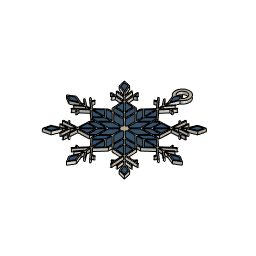
Snowflake 5 (Autodesk Fusion 360 design; units mm, degrees)
Autodesk Fusion 360 part; units mm, degrees
(part 1 of 2)
sketch "Sketch1" plane through (0, 0, 0) normal (0, 0, 1) x (1, 0, 0)
  line L0 (-4.9, 4.9) -> (4.9, 4.9)
  line L1 (4.9, 4.9) -> (4.9, -4.9)
  line L2 (4.9, -4.9) -> (-4.9, -4.9)
  line L3 (-4.9, -4.9) -> (-4.9, 4.9)
  line L4 (0, 4.9) -> (0, 0) construction
  line L5 (0, 0) -> (4.9, 0) construction
  dimension "d460" = 9.8
  constraint horizontal L0
  constraint vertical L1
  constraint vertical L3
  constraint horizontal L2
  constraint midpoint L0 L4.start
  constraint coincident L4.end L5.start
  constraint midpoint L1 L5.end
  constraint vertical L4
  constraint horizontal L5
  constraint equal L1 L2
  measures "d460" distance of L1.end L2.end
extrude "Extrude1" add sketch "Sketch1" along normal blind 5 makes body 1
sketch "Sketch2" plane through (0, 0, 0) normal (0, 0, 1) x (1, 0, 0)
  line L0 (-1.967, 4.9) -> (-0.9, 6.1716)
  line L1 (-0.9, 6.1716) -> (-0.9, 73.1716)
  line L2 (-0.9, 73.1716) -> (-6.182, 86.2449)
  line L3 (-6.182, 86.2449) -> (0, 96.4395)
  line L4 (0, 96.4395) -> (6.182, 86.2449)
  line L5 (6.182, 86.2449) -> (0.9, 73.1716)
  line L6 (0.9, 73.1716) -> (0.9, 6.1716)
  line L7 (0.9, 6.1716) -> (1.967, 4.9)
  line L8 (-4.2406, 86.2449) -> (0, 75.7491)
  line L9 (0, 75.7491) -> (4.2406, 86.2449)
  line L10 (4.2406, 86.2449) -> (0, 93.238)
  line L11 (0, 93.238) -> (-4.2406, 86.2449)
  line L12 (-4.9, 4.9) -> (4.9, 4.9) construction
  line L13 (0, 4.9) -> (0, 93.238) construction
  line L14 (-6.182, 86.2449) -> (6.182, 86.2449) construction
  line L15 (-1.967, 4.9) -> (1.967, 4.9)
  dimension "d463" = 1.8
  dimension "d464" = 80
  dimension "d465" = 1.66
  dimension "d466" = 1.8
  dimension "d468" = 158
  dimension "d469" = 14.1
  dimension "d470" = 67
  dimension "d471" = 1.66
  constraint coincident L7.end L12
  constraint coincident L0.start L12
  constraint midpoint L12 L13.start
  constraint vertical L13
  constraint vertical L3.end L10.end
  constraint coincident L8.end L13
  constraint coincident L8.start L14
  constraint coincident L9.end L14
  constraint horizontal L14
  constraint parallel L1 L6
  constraint symmetric L0 L7 L13
  constraint parallel L5 L9
  constraint parallel L2 L8
  constraint parallel L3 L11
  constraint parallel L4 L10
  constraint symmetric L8 L9 L13
  measures "d463" distance of L1 L6
  measures "d464" angle of L0 L7
  measures "d465" distance of L0.start L0.end
  measures "d466" distance of L5 L9
  measures "d468" angle of L5 L6
  measures "d469" distance of L4.end L5.end
  measures "d470" distance of L5.end L6.end
  measures "d471" distance of L4 L10
extrude "Extrude2" add sketch "Sketch2" along normal up to surface (5 mm away) bodies 1
sketch "Sketch3" plane through (0, 0, 0) normal (0, 0, 1) x (1, 0, 0)
  line L0 (0, 93.238) -> (-4.2406, 86.2449)
  line L1 (-4.2406, 86.2449) -> (0, 75.7491)
  line L2 (0, 75.7491) -> (4.2406, 86.2449)
  line L3 (4.2406, 86.2449) -> (0, 93.238)
  line L4 (4.9, -4.9) -> (-4.9, -4.9)
  line L5 (-4.9, -4.9) -> (-4.9, 4.9)
  line L6 (-4.9, 4.9) -> (-1.967, 4.9)
  line L7 (-1.967, 4.9) -> (-0.9, 6.1716)
  line L8 (-0.9, 6.1716) -> (-0.9, 73.1716)
  line L9 (-0.9, 73.1716) -> (-6.182, 86.2449)
  line L10 (-6.182, 86.2449) -> (0, 96.4395)
  line L11 (0, 96.4395) -> (6.182, 86.2449)
  line L12 (6.182, 86.2449) -> (0.9, 73.1716)
  line L13 (0.9, 73.1716) -> (0.9, 6.1716)
  line L14 (0.9, 6.1716) -> (1.967, 4.9)
  line L15 (1.967, 4.9) -> (4.9, 4.9)
  line L16 (4.9, 4.9) -> (4.9, -4.9)
  line L17 (0.9, 66.6716) -> (8.1032, 75.8914)
  line L18 (0.9, 63.7479) -> (9.5193, 74.7801)
  arc A0 (9.5193, 74.7801) -> (8.1008, 75.8883) centre (8.8101, 75.3342) ccw
  line L19 (0.9, 56.6479) -> (14.9397, 72.7987)
  line L20 (11.9485, 66.6141) -> (15.3003, 65.847)
  line L21 (10.6097, 65.074) -> (14.8988, 64.0923)
  line L22 (0.9, 53.9043) -> (10.6097, 65.074)
  line L23 (11.9485, 66.6141) -> (16.2982, 71.6178)
  arc A1 (14.8988, 64.0923) -> (15.3003, 65.847) centre (15.0995, 64.9697) ccw
  arc A2 (16.2982, 71.6178) -> (14.9397, 72.7987) centre (15.6189, 72.2083) ccw
  line L24 (1.8798, 55.0314) -> (14.4168, 41.1076)
  line L25 (14.4168, 41.1076) -> (14.4168, 13.4594)
  line L26 (14.4168, 13.4594) -> (4.9, 3.6044)
  line L27 (3.6489, 4.9) -> (12.6168, 14.1866)
  line L28 (0.9, 31.2992) -> (11.2116, 41.9773)
  line L29 (0.9, 33.8904) -> (10.0043, 43.3182)
  line L30 (0.9, 21.0447) -> (12.6168, 33.1778)
  line L31 (0.9, 18.4535) -> (12.6168, 30.5866)
  line L32 (12.6168, 14.1866) -> (12.6168, 30.5866)
  line L33 (12.6168, 33.1778) -> (12.6168, 40.4166)
  line L34 (12.6168, 40.4166) -> (11.2116, 41.9773)
  line L35 (10.0043, 43.3182) -> (0.9, 53.4295)
  line L36 (4.2635, 5.5365) -> (5.5365, 4.2635) construction
  dimension "d474" = 1.8
  dimension "d475" = 0.9
  dimension "d476" = 142
  dimension "d477" = 6.5
  dimension "d478" = 14
  dimension "d479" = 11.7
  dimension "d480" = 1.8
  dimension "d482" = 139
  dimension "d483" = 1.8
  dimension "d484" = 14.8
  dimension "d485" = 6.63
  dimension "d486" = 21.4
  dimension "d488" = 4.4
  dimension "d489" = 7.1
  dimension "d491" = 3.4385
  dimension "d492" = 1.8
  dimension "d493" = 45
  dimension "d494" = 13.7
  dimension "d495" = 1.8
  dimension "d496" = 1.8
  dimension "d497" = 1.8
  dimension "d498" = 1.8
  dimension "d499" = 97
  dimension "d500" = 136
  dimension "d502" = 16.4
  dimension "d503" = 2.1
  dimension "d504" = 18.7363
  constraint coincident L13 L17.start
  constraint coincident L13 L18.start
  constraint coincident L17.end A0
  constraint coincident L17 A0.end
  constraint parallel L17 L18
  constraint coincident L13 L19.start
  constraint coincident L13 L22.start
  constraint parallel L19 L22
  constraint coincident L20.start L22
  constraint parallel L20 L21
  constraint coincident L21.end A1
  constraint equal A0 A2
  constraint equal A1 A2
  constraint collinear L22 L23
  constraint coincident L21 A1.start
  constraint coincident L22 L24.start
  constraint vertical L25
  constraint coincident L16 L26.end
  constraint coincident L15 L27.start
  constraint coincident L13 L35.end
  constraint coincident L13 L28.start
  constraint coincident L13 L29.start
  constraint coincident L29.end L34
  constraint coincident L13 L30.start
  constraint coincident L30.end L32
  constraint coincident L13 L31.start
  constraint parallel L25 L32
  constraint parallel L28 L29
  constraint parallel L30 L31
  constraint parallel L26 L27
  constraint parallel L24 L34
  constraint parallel L24 L35
  constraint parallel L25 L33
  constraint coincident L27 L36.start
  constraint coincident L26 L36.end
  constraint midpoint L15.end L36
  constraint parallel L28 L31
  constraint parallel L26 L31
  measures "d474" distance of L17 L18
  measures "d475" radius of A0
  measures "d476" angle of L13 L18
  measures "d477" distance of L12.end L17.start
  measures "d478" distance of L18.start L18.end
  measures "d479" distance of L17.start L17.end
  measures "d480" distance of L19 L22
  measures "d482" angle of L13 L22
  measures "d483" distance of L20 L21
  measures "d484" distance of L22.start L21.start
  measures "d485" distance of L23.end L20.start
  measures "d486" distance of L19.start L19.end
  measures "d488" distance of L21.start L21.end
  measures "d489" distance of L18.start L19.start
  measures "d491" distance of L20.start L20.end
  measures "d492" distance of L26 L27
  measures "d493" angle of L15 L36
  measures "d494" distance of L25.end L26.end
  measures "d495" distance of L25 L32
  measures "d496" distance of L30 L31
  measures "d497" distance of L28 L29
  measures "d498" distance of L24 L35
  measures "d499" angle of L22 L24
  measures "d500" angle of L13 L28
  measures "d502" distance of L27.end L31.end
  measures "d503" distance of L33.end L28.end
  measures "d504" distance of L24.start L24.end
extrude "Extrude3" add sketch "Sketch3" along normal up to surface (5 mm away) contours L13 L15 L16 L22 L24 L25 L26 L27 L28 L29 L30 L31 L32 L33 L34 L35 | L13 L19 L20 L21 L22 L23 A1 A2 | L13 L17 L18 A0 bodies 1
mirror "Mirror1" about plane through (0, 0, 0) normal (1, 0, 0) of "Extrude3"
pattern_circular "C-Pattern1" count 8 over 360 about axis through (0, 0, 1.75) along (0, 0, 1) of bodies 1 makes body 2 at (-32.7449, 12.3565, 1.6667) makes body 3 at (-31.8915, 14.4168, 1.6667) makes body 4 at (-32.7449, -12.3565, 1.6667) makes body 5 at (-14.4168, -31.8915, 1.6667) makes body 6 at (12.3565, -32.7449, 1.6667) makes body 7 at (31.8915, -14.4168, 1.6667) makes body 8 at (12.3565, 32.7449, 1.6667)
combine "Combine1" operation add target body 1 tool bodies 2 7 8 6 5 4 3
sketch "Sketch4" plane through (0, 0, 0) normal (0, 0, 1) x (1, 0, 0)
  line L0 (-4.2635, -5.5365) -> (-12.4173, -13.98)
  line L1 (-12.4173, -13.98) -> (-12.6168, -25.4085)
  line L2 (-12.6168, -25.4085) -> (-12.6168, -30.4597)
  line L3 (-12.6168, -30.4597) -> (-9.0451, -26.888)
  line L4 (-9.0451, -26.888) -> (-1.105, -18.6658)
  line L5 (-1.105, -18.6658) -> (-0.9001, -6.9296)
  line L6 (-0.9001, -6.9296) -> (-0.9137, -6.1554)
  line L7 (-0.9137, -6.1554) -> (-1.6405, -5.2892)
  line L8 (-1.6405, -5.2892) -> (-2.0296, -4.9)
  line L9 (-2.0296, -4.9) -> (-2.58, -4.9)
  line L10 (-2.58, -4.9) -> (-3.7064, -4.9985)
  line L11 (-3.7064, -4.9985) -> (-4.2635, -5.5365)
  line L12 (-28.1497, -7.7612) -> (-21.2885, -0.9)
  line L13 (-21.2885, -0.9) -> (-31.2992, -0.9)
  line L14 (-31.2992, -0.9) -> (-41.9773, -11.2116)
  line L15 (-41.9773, -11.2116) -> (-40.4166, -12.6168)
  line L16 (-40.4166, -12.6168) -> (-33.1778, -12.6168)
  line L17 (-33.1778, -12.6168) -> (-28.1497, -7.7612)
  line L18 (-21.2885, 0.9) -> (-28.1497, 7.7612)
  line L19 (-28.1497, 7.7612) -> (-33.1778, 12.6168)
  line L20 (-33.1778, 12.6168) -> (-40.4166, 12.6168)
  line L21 (-40.4166, 12.6168) -> (-41.9773, 11.2116)
  line L22 (-41.9773, 11.2116) -> (-31.2992, 0.9)
  line L23 (-31.2992, 0.9) -> (-21.2885, 0.9)
  line L24 (-33.8904, 0.9) -> (-43.3182, 10.0043)
  line L25 (-43.3182, 10.0043) -> (-53.4295, 0.9)
  line L26 (-53.4295, 0.9) -> (-33.8904, 0.9)
  line L27 (-93.238, 0) -> (-86.2449, -4.2406)
  line L28 (-86.2449, -4.2406) -> (-75.7491, 0)
  line L29 (-75.7491, 0) -> (-86.2449, 4.2406)
  line L30 (-86.2449, 4.2406) -> (-93.238, 0)
  line L31 (-53.4295, -0.9) -> (-43.3182, -10.0043)
  line L32 (-43.3182, -10.0043) -> (-33.8904, -0.9)
  line L33 (-33.8904, -0.9) -> (-53.4295, -0.9)
  line L34 (-18.6658, -1.105) -> (-26.888, -9.0451)
  line L35 (-26.888, -9.0451) -> (-30.4597, -12.6168)
  line L36 (-30.4597, -12.6168) -> (-25.4085, -12.6168)
  line L37 (-25.4085, -12.6168) -> (-13.98, -12.4173)
  line L38 (-13.98, -12.4173) -> (-5.5365, -4.2635)
  line L39 (-5.5365, -4.2635) -> (-4.9985, -3.7064)
  line L40 (-4.9985, -3.7064) -> (-4.9, -2.58)
  line L41 (-4.9, -2.58) -> (-4.9, -2.0296)
  line L42 (-4.9, -2.0296) -> (-5.2892, -1.6405)
  line L43 (-5.2892, -1.6405) -> (-6.1554, -0.9137)
  line L44 (-6.1554, -0.9137) -> (-6.9296, -0.9001)
  line L45 (-6.9296, -0.9001) -> (-18.6658, -1.105)
  line L46 (-34.8053, -14.4168) -> (-41.1076, -14.4168)
  line L47 (-41.1076, -14.4168) -> (-55.0314, -1.8798)
  line L48 (-55.0314, -1.8798) -> (-65.074, -10.6097)
  line L49 (-65.074, -10.6097) -> (-64.0923, -14.8988)
  arc A0 (-65.847, -15.3003) -> (-64.0923, -14.8988) centre (-64.9697, -15.0995) ccw
  line L50 (-65.847, -15.3003) -> (-66.6141, -11.9485)
  line L51 (-66.6141, -11.9485) -> (-71.6178, -16.2982)
  arc A1 (-72.7987, -14.9397) -> (-71.6178, -16.2982) centre (-72.2083, -15.6189) ccw
  line L52 (-72.7987, -14.9397) -> (-56.6479, -0.9)
  line L53 (-56.6479, -0.9) -> (-63.7479, -0.9)
  line L54 (-63.7479, -0.9) -> (-74.7801, -9.5193)
  arc A2 (-75.8883, -8.1008) -> (-74.7801, -9.5193) centre (-75.3342, -8.8101) ccw
  line L55 (-75.8883, -8.1008) -> (-66.6716, -0.9)
  line L56 (-66.6716, -0.9) -> (-73.1716, -0.9)
  line L57 (-73.1716, -0.9) -> (-86.2449, -6.182)
  line L58 (-86.2449, -6.182) -> (-96.4395, 0)
  line L59 (-96.4395, 0) -> (-86.2449, 6.182)
  line L60 (-86.2449, 6.182) -> (-73.1716, 0.9)
  line L61 (-73.1716, 0.9) -> (-66.6716, 0.9)
  line L62 (-66.6716, 0.9) -> (-75.8883, 8.1008)
  arc A3 (-74.7801, 9.5193) -> (-75.8883, 8.1008) centre (-75.3342, 8.8101) ccw
  line L63 (-74.7801, 9.5193) -> (-63.7479, 0.9)
  line L64 (-63.7479, 0.9) -> (-56.6479, 0.9)
  line L65 (-56.6479, 0.9) -> (-72.7987, 14.9397)
  arc A4 (-71.6178, 16.2982) -> (-72.7987, 14.9397) centre (-72.2083, 15.6189) ccw
  line L66 (-71.6178, 16.2982) -> (-66.6141, 11.9485)
  line L67 (-66.6141, 11.9485) -> (-65.847, 15.3003)
  arc A5 (-64.0923, 14.8988) -> (-65.847, 15.3003) centre (-64.9697, 15.0995) ccw
  line L68 (-64.0923, 14.8988) -> (-65.074, 10.6097)
  line L69 (-65.074, 10.6097) -> (-55.0314, 1.8798)
  line L70 (-55.0314, 1.8798) -> (-41.1076, 14.4168)
  line L71 (-41.1076, 14.4168) -> (-34.8053, 14.4168)
  line L72 (-34.8053, 14.4168) -> (-39.2617, 18.8732)
  line L73 (-39.2617, 18.8732) -> (-40.2423, 37.5839)
  line L74 (-40.2423, 37.5839) -> (-53.5164, 38.5121)
  line L75 (-53.5164, 38.5121) -> (-55.8551, 34.7851)
  arc A6 (-57.3798, 35.7419) -> (-55.8551, 34.7851) centre (-56.6175, 35.2635) ccw
  line L76 (-57.3798, 35.7419) -> (-55.5521, 38.6544)
  line L77 (-55.5521, 38.6544) -> (-62.166, 39.1169)
  arc A7 (-62.0404, 40.9125) -> (-62.166, 39.1169) centre (-62.1032, 40.0147) ccw
  line L78 (-62.0404, 40.9125) -> (-40.6925, 39.4198)
  line L79 (-40.6925, 39.4198) -> (-45.713, 44.4402)
  line L80 (-45.713, 44.4402) -> (-59.6086, 46.1464)
  arc A8 (-59.3893, 47.933) -> (-59.6086, 46.1464) centre (-59.499, 47.0397) ccw
  line L81 (-59.3893, 47.933) -> (-47.7804, 46.5076)
  line L82 (-47.7804, 46.5076) -> (-52.3766, 51.1038)
  line L83 (-52.3766, 51.1038) -> (-65.3557, 56.6131)
  line L84 (-65.3557, 56.6131) -> (-68.193, 68.193)
  line L85 (-68.193, 68.193) -> (-56.6131, 65.3557)
  line L86 (-56.6131, 65.3557) -> (-51.1038, 52.3766)
  line L87 (-51.1038, 52.3766) -> (-46.5076, 47.7804)
  line L88 (-46.5076, 47.7804) -> (-47.933, 59.3893)
  arc A9 (-46.1464, 59.6086) -> (-47.933, 59.3893) centre (-47.0397, 59.499) ccw
  line L89 (-46.1464, 59.6086) -> (-44.4402, 45.713)
  line L90 (-44.4402, 45.713) -> (-39.4198, 40.6925)
  line L91 (-39.4198, 40.6925) -> (-40.9125, 62.0404)
  arc A10 (-39.1169, 62.166) -> (-40.9125, 62.0404) centre (-40.0147, 62.1032) ccw
  line L92 (-39.1169, 62.166) -> (-38.6544, 55.5521)
  line L93 (-38.6544, 55.5521) -> (-35.7419, 57.3798)
  arc A11 (-34.7851, 55.8551) -> (-35.7419, 57.3798) centre (-35.2635, 56.6175) ccw
  line L94 (-34.7851, 55.8551) -> (-38.5121, 53.5164)
  line L95 (-38.5121, 53.5164) -> (-37.5839, 40.2423)
  line L96 (-37.5839, 40.2423) -> (-18.8732, 39.2617)
  line L97 (-18.8732, 39.2617) -> (-14.4168, 34.8053)
  line L98 (-14.4168, 34.8053) -> (-14.4168, 41.1076)
  line L99 (-14.4168, 41.1076) -> (-1.8798, 55.0314)
  line L100 (-1.8798, 55.0314) -> (-10.6097, 65.074)
  line L101 (-10.6097, 65.074) -> (-14.8988, 64.0923)
  arc A12 (-15.3003, 65.847) -> (-14.8988, 64.0923) centre (-15.0995, 64.9697) ccw
  line L102 (-15.3003, 65.847) -> (-11.9485, 66.6141)
  line L103 (-11.9485, 66.6141) -> (-16.2982, 71.6178)
  arc A13 (-14.9397, 72.7987) -> (-16.2982, 71.6178) centre (-15.6189, 72.2083) ccw
  line L104 (-14.9397, 72.7987) -> (-0.9, 56.6479)
  line L105 (-0.9, 56.6479) -> (-0.9, 63.7479)
  line L106 (-0.9, 63.7479) -> (-9.5193, 74.7801)
  arc A14 (-8.1008, 75.8883) -> (-9.5193, 74.7801) centre (-8.8101, 75.3342) ccw
  line L107 (-8.1008, 75.8883) -> (-0.9, 66.6716)
  line L108 (-0.9, 66.6716) -> (-0.9, 73.1716)
  line L109 (-0.9, 73.1716) -> (-6.182, 86.2449)
  line L110 (-6.182, 86.2449) -> (0, 96.4395)
  line L111 (0, 96.4395) -> (6.182, 86.2449)
  line L112 (6.182, 86.2449) -> (0.9, 73.1716)
  line L113 (0.9, 73.1716) -> (0.9, 66.6716)
  line L114 (0.9, 66.6716) -> (8.1008, 75.8883)
  arc A15 (9.5193, 74.7801) -> (8.1008, 75.8883) centre (8.8101, 75.3342) ccw
  line L115 (9.5193, 74.7801) -> (0.9, 63.7479)
  line L116 (0.9, 63.7479) -> (0.9, 56.6479)
  line L117 (0.9, 56.6479) -> (14.9397, 72.7987)
  arc A16 (16.2982, 71.6178) -> (14.9397, 72.7987) centre (15.6189, 72.2083) ccw
  line L118 (16.2982, 71.6178) -> (11.9485, 66.6141)
  line L119 (11.9485, 66.6141) -> (15.3003, 65.847)
  arc A17 (14.8988, 64.0923) -> (15.3003, 65.847) centre (15.0995, 64.9697) ccw
  line L120 (14.8988, 64.0923) -> (10.6097, 65.074)
  line L121 (10.6097, 65.074) -> (1.8798, 55.0314)
  line L122 (1.8798, 55.0314) -> (14.4168, 41.1076)
  line L123 (14.4168, 41.1076) -> (14.4168, 34.8053)
  line L124 (14.4168, 34.8053) -> (18.8732, 39.2617)
  line L125 (18.8732, 39.2617) -> (37.5839, 40.2423)
  line L126 (37.5839, 40.2423) -> (38.5121, 53.5164)
  line L127 (38.5121, 53.5164) -> (34.7851, 55.8551)
  arc A18 (35.7419, 57.3798) -> (34.7851, 55.8551) centre (35.2635, 56.6175) ccw
  line L128 (35.7419, 57.3798) -> (38.6544, 55.5521)
  line L129 (38.6544, 55.5521) -> (39.1169, 62.166)
  arc A19 (40.9125, 62.0404) -> (39.1169, 62.166) centre (40.0147, 62.1032) ccw
  line L130 (40.9125, 62.0404) -> (39.4198, 40.6925)
  line L131 (39.4198, 40.6925) -> (44.4402, 45.713)
  line L132 (44.4402, 45.713) -> (46.1464, 59.6086)
  arc A20 (47.933, 59.3893) -> (46.1464, 59.6086) centre (47.0397, 59.499) ccw
  line L133 (47.933, 59.3893) -> (46.5076, 47.7804)
  line L134 (46.5076, 47.7804) -> (51.1038, 52.3766)
  line L135 (51.1038, 52.3766) -> (56.6131, 65.3557)
  line L136 (56.6131, 65.3557) -> (68.193, 68.193)
  line L137 (68.193, 68.193) -> (65.3557, 56.6131)
  line L138 (65.3557, 56.6131) -> (52.3766, 51.1038)
  line L139 (52.3766, 51.1038) -> (47.7804, 46.5076)
  line L140 (47.7804, 46.5076) -> (59.3893, 47.933)
  arc A21 (59.6086, 46.1464) -> (59.3893, 47.933) centre (59.499, 47.0397) ccw
  line L141 (59.6086, 46.1464) -> (45.713, 44.4402)
  line L142 (45.713, 44.4402) -> (40.6925, 39.4198)
  line L143 (40.6925, 39.4198) -> (62.0404, 40.9125)
  arc A22 (62.166, 39.1169) -> (62.0404, 40.9125) centre (62.1032, 40.0147) ccw
  line L144 (62.166, 39.1169) -> (55.5521, 38.6544)
  line L145 (55.5521, 38.6544) -> (57.3798, 35.7419)
  arc A23 (55.8551, 34.7851) -> (57.3798, 35.7419) centre (56.6175, 35.2635) ccw
  line L146 (55.8551, 34.7851) -> (53.5164, 38.5121)
  line L147 (53.5164, 38.5121) -> (40.2423, 37.5839)
  line L148 (40.2423, 37.5839) -> (39.2617, 18.8732)
  line L149 (39.2617, 18.8732) -> (34.8053, 14.4168)
  line L150 (34.8053, 14.4168) -> (41.1076, 14.4168)
  line L151 (41.1076, 14.4168) -> (55.0314, 1.8798)
  line L152 (55.0314, 1.8798) -> (65.074, 10.6097)
  line L153 (65.074, 10.6097) -> (64.0923, 14.8988)
  arc A24 (65.847, 15.3003) -> (64.0923, 14.8988) centre (64.9697, 15.0995) ccw
  line L154 (65.847, 15.3003) -> (66.6141, 11.9485)
  line L155 (66.6141, 11.9485) -> (71.6178, 16.2982)
  arc A25 (72.7987, 14.9397) -> (71.6178, 16.2982) centre (72.2083, 15.6189) ccw
  line L156 (72.7987, 14.9397) -> (56.6479, 0.9)
  line L157 (56.6479, 0.9) -> (63.7479, 0.9)
  line L158 (63.7479, 0.9) -> (74.7801, 9.5193)
  arc A26 (75.8883, 8.1008) -> (74.7801, 9.5193) centre (75.3342, 8.8101) ccw
  line L159 (75.8883, 8.1008) -> (66.6716, 0.9)
  line L160 (66.6716, 0.9) -> (73.1716, 0.9)
  line L161 (73.1716, 0.9) -> (86.2449, 6.182)
  line L162 (86.2449, 6.182) -> (96.4395, 0)
  line L163 (96.4395, 0) -> (86.2449, -6.182)
  line L164 (86.2449, -6.182) -> (73.1716, -0.9)
  line L165 (73.1716, -0.9) -> (66.6716, -0.9)
  line L166 (66.6716, -0.9) -> (75.8883, -8.1008)
  arc A27 (74.7801, -9.5193) -> (75.8883, -8.1008) centre (75.3342, -8.8101) ccw
  line L167 (74.7801, -9.5193) -> (63.7479, -0.9)
  line L168 (63.7479, -0.9) -> (56.6479, -0.9)
  line L169 (56.6479, -0.9) -> (72.7987, -14.9397)
  arc A28 (71.6178, -16.2982) -> (72.7987, -14.9397) centre (72.2083, -15.6189) ccw
  line L170 (71.6178, -16.2982) -> (66.6141, -11.9485)
  line L171 (66.6141, -11.9485) -> (65.847, -15.3003)
  arc A29 (64.0923, -14.8988) -> (65.847, -15.3003) centre (64.9697, -15.0995) ccw
  line L172 (64.0923, -14.8988) -> (65.074, -10.6097)
  line L173 (65.074, -10.6097) -> (55.0314, -1.8798)
  line L174 (55.0314, -1.8798) -> (41.1076, -14.4168)
  line L175 (41.1076, -14.4168) -> (34.8053, -14.4168)
  line L176 (34.8053, -14.4168) -> (39.2617, -18.8732)
  line L177 (39.2617, -18.8732) -> (40.2423, -37.5839)
  line L178 (40.2423, -37.5839) -> (53.5164, -38.5121)
  line L179 (53.5164, -38.5121) -> (55.8551, -34.7851)
  arc A30 (57.3798, -35.7419) -> (55.8551, -34.7851) centre (56.6175, -35.2635) ccw
  line L180 (57.3798, -35.7419) -> (55.5521, -38.6544)
  line L181 (55.5521, -38.6544) -> (62.166, -39.1169)
  arc A31 (62.0404, -40.9125) -> (62.166, -39.1169) centre (62.1032, -40.0147) ccw
  line L182 (62.0404, -40.9125) -> (40.6925, -39.4198)
  line L183 (40.6925, -39.4198) -> (45.713, -44.4402)
  line L184 (45.713, -44.4402) -> (59.6086, -46.1464)
  arc A32 (59.3893, -47.933) -> (59.6086, -46.1464) centre (59.499, -47.0397) ccw
  line L185 (59.3893, -47.933) -> (47.7804, -46.5076)
  line L186 (47.7804, -46.5076) -> (52.3766, -51.1038)
  line L187 (52.3766, -51.1038) -> (65.3557, -56.6131)
  line L188 (65.3557, -56.6131) -> (68.193, -68.193)
  line L189 (68.193, -68.193) -> (56.6131, -65.3557)
  line L190 (56.6131, -65.3557) -> (51.1038, -52.3766)
  line L191 (51.1038, -52.3766) -> (46.5076, -47.7804)
  line L192 (46.5076, -47.7804) -> (47.933, -59.3893)
  arc A33 (46.1464, -59.6086) -> (47.933, -59.3893) centre (47.0397, -59.499) ccw
  line L193 (46.1464, -59.6086) -> (44.4402, -45.713)
  line L194 (44.4402, -45.713) -> (39.4198, -40.6925)
  line L195 (39.4198, -40.6925) -> (40.9125, -62.0404)
  arc A34 (39.1169, -62.166) -> (40.9125, -62.0404) centre (40.0147, -62.1032) ccw
  line L196 (39.1169, -62.166) -> (38.6544, -55.5521)
  line L197 (38.6544, -55.5521) -> (35.7419, -57.3798)
  arc A35 (34.7851, -55.8551) -> (35.7419, -57.3798) centre (35.2635, -56.6175) ccw
  line L198 (34.7851, -55.8551) -> (38.5121, -53.5164)
  line L199 (38.5121, -53.5164) -> (37.5839, -40.2423)
  line L200 (37.5839, -40.2423) -> (18.8732, -39.2617)
  line L201 (18.8732, -39.2617) -> (14.4168, -34.8053)
  line L202 (14.4168, -34.8053) -> (14.4168, -41.1076)
  line L203 (14.4168, -41.1076) -> (1.8798, -55.0314)
  line L204 (1.8798, -55.0314) -> (10.6097, -65.074)
  line L205 (10.6097, -65.074) -> (14.8988, -64.0923)
  arc A36 (15.3003, -65.847) -> (14.8988, -64.0923) centre (15.0995, -64.9697) ccw
  line L206 (15.3003, -65.847) -> (11.9485, -66.6141)
  line L207 (11.9485, -66.6141) -> (16.2982, -71.6178)
  arc A37 (14.9397, -72.7987) -> (16.2982, -71.6178) centre (15.6189, -72.2083) ccw
  line L208 (14.9397, -72.7987) -> (0.9, -56.6479)
  line L209 (0.9, -56.6479) -> (0.9, -63.7479)
  line L210 (0.9, -63.7479) -> (9.5193, -74.7801)
  arc A38 (8.1008, -75.8883) -> (9.5193, -74.7801) centre (8.8101, -75.3342) ccw
  line L211 (8.1008, -75.8883) -> (0.9, -66.6716)
  line L212 (0.9, -66.6716) -> (0.9, -73.1716)
  line L213 (0.9, -73.1716) -> (6.182, -86.2449)
  line L214 (6.182, -86.2449) -> (0, -96.4395)
  line L215 (0, -96.4395) -> (-6.182, -86.2449)
  line L216 (-6.182, -86.2449) -> (-0.9, -73.1716)
  line L217 (-0.9, -73.1716) -> (-0.9, -66.6716)
  line L218 (-0.9, -66.6716) -> (-8.1008, -75.8883)
  arc A39 (-9.5193, -74.7801) -> (-8.1008, -75.8883) centre (-8.8101, -75.3342) ccw
  line L219 (-9.5193, -74.7801) -> (-0.9, -63.7479)
  line L220 (-0.9, -63.7479) -> (-0.9, -56.6479)
  line L221 (-0.9, -56.6479) -> (-14.9397, -72.7987)
  arc A40 (-16.2982, -71.6178) -> (-14.9397, -72.7987) centre (-15.6189, -72.2083) ccw
  line L222 (-16.2982, -71.6178) -> (-11.9485, -66.6141)
  line L223 (-11.9485, -66.6141) -> (-15.3003, -65.847)
  arc A41 (-14.8988, -64.0923) -> (-15.3003, -65.847) centre (-15.0995, -64.9697) ccw
  line L224 (-14.8988, -64.0923) -> (-10.6097, -65.074)
  line L225 (-10.6097, -65.074) -> (-1.8798, -55.0314)
  line L226 (-1.8798, -55.0314) -> (-14.4168, -41.1076)
  line L227 (-14.4168, -41.1076) -> (-14.4168, -34.8053)
  line L228 (-14.4168, -34.8053) -> (-18.8732, -39.2617)
  line L229 (-18.8732, -39.2617) -> (-37.5839, -40.2423)
  line L230 (-37.5839, -40.2423) -> (-38.5121, -53.5164)
  line L231 (-38.5121, -53.5164) -> (-34.7851, -55.8551)
  arc A42 (-35.7419, -57.3798) -> (-34.7851, -55.8551) centre (-35.2635, -56.6175) ccw
  line L232 (-35.7419, -57.3798) -> (-38.6544, -55.5521)
  line L233 (-38.6544, -55.5521) -> (-39.1169, -62.166)
  arc A43 (-40.9125, -62.0404) -> (-39.1169, -62.166) centre (-40.0147, -62.1032) ccw
  line L234 (-40.9125, -62.0404) -> (-39.4198, -40.6925)
  line L235 (-39.4198, -40.6925) -> (-44.4402, -45.713)
  line L236 (-44.4402, -45.713) -> (-46.1464, -59.6086)
  arc A44 (-47.933, -59.3893) -> (-46.1464, -59.6086) centre (-47.0397, -59.499) ccw
  line L237 (-47.933, -59.3893) -> (-46.5076, -47.7804)
  line L238 (-46.5076, -47.7804) -> (-51.1038, -52.3766)
  line L239 (-51.1038, -52.3766) -> (-56.6131, -65.3557)
  line L240 (-56.6131, -65.3557) -> (-68.193, -68.193)
  line L241 (-68.193, -68.193) -> (-65.3557, -56.6131)
  line L242 (-65.3557, -56.6131) -> (-52.3766, -51.1038)
  line L243 (-52.3766, -51.1038) -> (-47.7804, -46.5076)
  line L244 (-47.7804, -46.5076) -> (-59.3893, -47.933)
  arc A45 (-59.6086, -46.1464) -> (-59.3893, -47.933) centre (-59.499, -47.0397) ccw
  line L245 (-59.6086, -46.1464) -> (-45.713, -44.4402)
  line L246 (-45.713, -44.4402) -> (-40.6925, -39.4198)
  line L247 (-40.6925, -39.4198) -> (-62.0404, -40.9125)
  arc A46 (-62.166, -39.1169) -> (-62.0404, -40.9125) centre (-62.1032, -40.0147) ccw
  line L248 (-62.166, -39.1169) -> (-55.5521, -38.6544)
  line L249 (-55.5521, -38.6544) -> (-57.3798, -35.7419)
  arc A47 (-55.8551, -34.7851) -> (-57.3798, -35.7419) centre (-56.6175, -35.2635) ccw
  line L250 (-55.8551, -34.7851) -> (-53.5164, -38.5121)
  line L251 (-53.5164, -38.5121) -> (-40.2423, -37.5839)
  line L252 (-40.2423, -37.5839) -> (-39.2617, -18.8732)
  line L253 (-39.2617, -18.8732) -> (-34.8053, -14.4168)
  line L254 (4.9, 2.0296) -> (5.2892, 1.6405)
  line L255 (5.2892, 1.6405) -> (6.1554, 0.9137)
  line L256 (6.1554, 0.9137) -> (6.9296, 0.9001)
  line L257 (6.9296, 0.9001) -> (18.6658, 1.105)
  line L258 (18.6658, 1.105) -> (26.888, 9.0451)
  line L259 (26.888, 9.0451) -> (30.4597, 12.6168)
  line L260 (30.4597, 12.6168) -> (25.4085, 12.6168)
  line L261 (25.4085, 12.6168) -> (13.98, 12.4173)
  line L262 (13.98, 12.4173) -> (5.5365, 4.2635)
  line L263 (5.5365, 4.2635) -> (4.9985, 3.7064)
  line L264 (4.9985, 3.7064) -> (4.9, 2.58)
  line L265 (4.9, 2.58) -> (4.9, 2.0296)
  line L266 (-25.3928, 14.4168) -> (-15.6896, 14.4168)
  line L267 (-15.6896, 14.4168) -> (-22.7683, 21.4955)
  line L268 (-22.7683, 21.4955) -> (-37.6102, 21.7546)
  line L269 (-37.6102, 21.7546) -> (-37.5003, 19.6574)
  line L270 (-37.5003, 19.6574) -> (-32.3817, 14.5388)
  line L271 (-32.3817, 14.5388) -> (-25.3928, 14.4168)
  line L272 (-14.4168, -15.6896) -> (-21.4955, -22.7683)
  line L273 (-21.4955, -22.7683) -> (-21.7546, -37.6102)
  line L274 (-21.7546, -37.6102) -> (-19.6574, -37.5003)
  line L275 (-19.6574, -37.5003) -> (-14.5388, -32.3817)
  line L276 (-14.5388, -32.3817) -> (-14.4168, -25.3928)
  line L277 (-14.4168, -25.3928) -> (-14.4168, -15.6896)
  line L278 (28.1497, -7.7612) -> (33.1778, -12.6168)
  line L279 (33.1778, -12.6168) -> (40.4166, -12.6168)
  line L280 (40.4166, -12.6168) -> (41.9773, -11.2116)
  line L281 (41.9773, -11.2116) -> (31.2992, -0.9)
  line L282 (31.2992, -0.9) -> (21.2885, -0.9)
  line L283 (21.2885, -0.9) -> (28.1497, -7.7612)
  line L284 (14.4168, 25.3928) -> (14.4168, 15.6896)
  line L285 (14.4168, 15.6896) -> (21.4955, 22.7683)
  line L286 (21.4955, 22.7683) -> (21.7546, 37.6102)
  line L287 (21.7546, 37.6102) -> (19.6574, 37.5003)
  line L288 (19.6574, 37.5003) -> (14.5388, 32.3817)
  line L289 (14.5388, 32.3817) -> (14.4168, 25.3928)
  line L290 (15.6896, 14.4168) -> (25.3928, 14.4168)
  line L291 (25.3928, 14.4168) -> (32.3817, 14.5388)
  line L292 (32.3817, 14.5388) -> (37.5003, 19.6574)
  line L293 (37.5003, 19.6574) -> (37.6102, 21.7546)
  line L294 (37.6102, 21.7546) -> (22.7683, 21.4955)
  line L295 (22.7683, 21.4955) -> (15.6896, 14.4168)
  line L296 (24.6006, 23.3278) -> (37.7047, 23.5565)
  line L297 (37.7047, 23.5565) -> (38.4168, 37.144)
  line L298 (38.4168, 37.144) -> (24.6006, 23.3278)
  line L299 (65.9292, 65.9292) -> (57.9858, 63.9829)
  line L300 (57.9858, 63.9829) -> (53.5627, 53.5627)
  line L301 (53.5627, 53.5627) -> (63.9829, 57.9858)
  line L302 (63.9829, 57.9858) -> (65.9292, 65.9292)
  line L303 (37.144, 38.4168) -> (23.5565, 37.7047)
  line L304 (23.5565, 37.7047) -> (23.3278, 24.6006)
  line L305 (23.3278, 24.6006) -> (37.144, 38.4168)
  line L306 (7.7612, 28.1497) -> (12.6168, 33.1778)
  line L307 (12.6168, 33.1778) -> (12.6168, 40.4166)
  line L308 (12.6168, 40.4166) -> (11.2116, 41.9773)
  line L309 (11.2116, 41.9773) -> (0.9, 31.2992)
  line L310 (0.9, 31.2992) -> (0.9, 21.2885)
  line L311 (0.9, 21.2885) -> (7.7612, 28.1497)
  line L312 (0.9, 33.8904) -> (10.0043, 43.3182)
  line L313 (10.0043, 43.3182) -> (0.9, 53.4295)
  line L314 (0.9, 53.4295) -> (0.9, 33.8904)
  line L315 (0, 93.238) -> (-4.2406, 86.2449)
  line L316 (-4.2406, 86.2449) -> (0, 75.7491)
  line L317 (0, 75.7491) -> (4.2406, 86.2449)
  line L318 (4.2406, 86.2449) -> (0, 93.238)
  line L319 (-0.9, 53.4295) -> (-10.0043, 43.3182)
  line L320 (-10.0043, 43.3182) -> (-0.9, 33.8904)
  line L321 (-0.9, 33.8904) -> (-0.9, 53.4295)
  line L322 (-7.7612, 28.1497) -> (-0.9, 21.2885)
  line L323 (-0.9, 21.2885) -> (-0.9, 31.2992)
  line L324 (-0.9, 31.2992) -> (-11.2116, 41.9773)
  line L325 (-11.2116, 41.9773) -> (-12.6168, 40.4166)
  line L326 (-12.6168, 40.4166) -> (-12.6168, 33.1778)
  line L327 (-12.6168, 33.1778) -> (-7.7612, 28.1497)
  line L328 (-23.3278, 24.6006) -> (-23.5565, 37.7047)
  line L329 (-23.5565, 37.7047) -> (-37.144, 38.4168)
  line L330 (-37.144, 38.4168) -> (-23.3278, 24.6006)
  line L331 (-65.9292, 65.9292) -> (-63.9829, 57.9858)
  line L332 (-63.9829, 57.9858) -> (-53.5627, 53.5627)
  line L333 (-53.5627, 53.5627) -> (-57.9858, 63.9829)
  line L334 (-57.9858, 63.9829) -> (-65.9292, 65.9292)
  line L335 (-38.4168, 37.144) -> (-37.7047, 23.5565)
  line L336 (-37.7047, 23.5565) -> (-24.6006, 23.3278)
  line L337 (-24.6006, 23.3278) -> (-38.4168, 37.144)
  line L338 (-14.4168, 25.3928) -> (-14.5388, 32.3817)
  line L339 (-14.5388, 32.3817) -> (-19.6574, 37.5003)
  line L340 (-19.6574, 37.5003) -> (-21.7546, 37.6102)
  line L341 (-21.7546, 37.6102) -> (-21.4955, 22.7683)
  line L342 (-21.4955, 22.7683) -> (-14.4168, 15.6896)
  line L343 (-14.4168, 15.6896) -> (-14.4168, 25.3928)
  line L344 (53.4295, 0.9) -> (43.3182, 10.0043)
  line L345 (43.3182, 10.0043) -> (33.8904, 0.9)
  line L346 (33.8904, 0.9) -> (53.4295, 0.9)
  line L347 (93.238, 0) -> (86.2449, 4.2406)
  line L348 (86.2449, 4.2406) -> (75.7491, 0)
  line L349 (75.7491, 0) -> (86.2449, -4.2406)
  line L350 (86.2449, -4.2406) -> (93.238, 0)
  line L351 (33.8904, -0.9) -> (43.3182, -10.0043)
  line L352 (43.3182, -10.0043) -> (53.4295, -0.9)
  line L353 (53.4295, -0.9) -> (33.8904, -0.9)
  line L354 (28.1497, 7.7612) -> (21.2885, 0.9)
  line L355 (21.2885, 0.9) -> (31.2992, 0.9)
  line L356 (31.2992, 0.9) -> (41.9773, 11.2116)
  line L357 (41.9773, 11.2116) -> (40.4166, 12.6168)
  line L358 (40.4166, 12.6168) -> (33.1778, 12.6168)
  line L359 (33.1778, 12.6168) -> (28.1497, 7.7612)
  line L360 (23.3278, -24.6006) -> (23.5565, -37.7047)
  line L361 (23.5565, -37.7047) -> (37.144, -38.4168)
  line L362 (37.144, -38.4168) -> (23.3278, -24.6006)
  line L363 (65.9292, -65.9292) -> (63.9829, -57.9858)
  line L364 (63.9829, -57.9858) -> (53.5627, -53.5627)
  line L365 (53.5627, -53.5627) -> (57.9858, -63.9829)
  line L366 (57.9858, -63.9829) -> (65.9292, -65.9292)
  line L367 (38.4168, -37.144) -> (37.7047, -23.5565)
  line L368 (37.7047, -23.5565) -> (24.6006, -23.3278)
  line L369 (24.6006, -23.3278) -> (38.4168, -37.144)
  line L370 (15.6896, -14.4168) -> (22.7683, -21.4955)
  line L371 (22.7683, -21.4955) -> (37.6102, -21.7546)
  line L372 (37.6102, -21.7546) -> (37.5003, -19.6574)
  line L373 (37.5003, -19.6574) -> (32.3817, -14.5388)
  line L374 (32.3817, -14.5388) -> (25.3928, -14.4168)
  line L375 (25.3928, -14.4168) -> (15.6896, -14.4168)
  line L376 (14.4168, -25.3928) -> (14.5388, -32.3817)
  line L377 (14.5388, -32.3817) -> (19.6574, -37.5003)
  line L378 (19.6574, -37.5003) -> (21.7546, -37.6102)
  line L379 (21.7546, -37.6102) -> (21.4955, -22.7683)
  line L380 (21.4955, -22.7683) -> (14.4168, -15.6896)
  line L381 (14.4168, -15.6896) -> (14.4168, -25.3928)
  line L382 (0.9, -21.2885) -> (0.9, -31.2992)
  line L383 (0.9, -31.2992) -> (11.2116, -41.9773)
  line L384 (11.2116, -41.9773) -> (12.6168, -40.4166)
  line L385 (12.6168, -40.4166) -> (12.6168, -33.1778)
  line L386 (12.6168, -33.1778) -> (7.7612, -28.1497)
  line L387 (7.7612, -28.1497) -> (0.9, -21.2885)
  line L388 (-0.9, -33.8904) -> (-10.0043, -43.3182)
  line L389 (-10.0043, -43.3182) -> (-0.9, -53.4295)
  line L390 (-0.9, -53.4295) -> (-0.9, -33.8904)
  line L391 (0, -93.238) -> (4.2406, -86.2449)
  line L392 (4.2406, -86.2449) -> (0, -75.7491)
  line L393 (0, -75.7491) -> (-4.2406, -86.2449)
  line L394 (-4.2406, -86.2449) -> (0, -93.238)
  line L395 (0.9, -53.4295) -> (10.0043, -43.3182)
  line L396 (10.0043, -43.3182) -> (0.9, -33.8904)
  line L397 (0.9, -33.8904) -> (0.9, -53.4295)
  line L398 (-7.7612, -28.1497) -> (-12.6168, -33.1778)
  line L399 (-12.6168, -33.1778) -> (-12.6168, -40.4166)
  line L400 (-12.6168, -40.4166) -> (-11.2116, -41.9773)
  line L401 (-11.2116, -41.9773) -> (-0.9, -31.2992)
  line L402 (-0.9, -31.2992) -> (-0.9, -21.2885)
  line L403 (-0.9, -21.2885) -> (-7.7612, -28.1497)
  line L404 (-37.144, -38.4168) -> (-23.5565, -37.7047)
  line L405 (-23.5565, -37.7047) -> (-23.3278, -24.6006)
  line L406 (-23.3278, -24.6006) -> (-37.144, -38.4168)
  line L407 (-65.9292, -65.9292) -> (-57.9858, -63.9829)
  line L408 (-57.9858, -63.9829) -> (-53.5627, -53.5627)
  line L409 (-53.5627, -53.5627) -> (-63.9829, -57.9858)
  line L410 (-63.9829, -57.9858) -> (-65.9292, -65.9292)
  line L411 (-24.6006, -23.3278) -> (-37.7047, -23.5565)
  line L412 (-37.7047, -23.5565) -> (-38.4168, -37.144)
  line L413 (-38.4168, -37.144) -> (-24.6006, -23.3278)
  line L414 (-2.0296, 4.9) -> (-1.6405, 5.2892)
  line L415 (-1.6405, 5.2892) -> (-0.9137, 6.1554)
  line L416 (-0.9137, 6.1554) -> (-0.9001, 6.9296)
  line L417 (-0.9001, 6.9296) -> (-1.105, 18.6658)
  line L418 (-1.105, 18.6658) -> (-9.0451, 26.888)
  line L419 (-9.0451, 26.888) -> (-12.6168, 30.4597)
  line L420 (-12.6168, 30.4597) -> (-12.6168, 25.4085)
  line L421 (-12.6168, 25.4085) -> (-12.4173, 13.98)
  line L422 (-12.4173, 13.98) -> (-4.2635, 5.5365)
  line L423 (-4.2635, 5.5365) -> (-3.7064, 4.9985)
  line L424 (-3.7064, 4.9985) -> (-2.58, 4.9)
  line L425 (-2.58, 4.9) -> (-2.0296, 4.9)
  line L426 (2.58, 4.9) -> (3.7064, 4.9985)
  line L427 (3.7064, 4.9985) -> (4.2635, 5.5365)
  line L428 (4.2635, 5.5365) -> (12.4173, 13.98)
  line L429 (12.4173, 13.98) -> (12.6168, 25.4085)
  line L430 (12.6168, 25.4085) -> (12.6168, 30.4597)
  line L431 (12.6168, 30.4597) -> (9.0451, 26.888)
  line L432 (9.0451, 26.888) -> (1.105, 18.6658)
  line L433 (1.105, 18.6658) -> (0.9001, 6.9296)
  line L434 (0.9001, 6.9296) -> (0.9137, 6.1554)
  line L435 (0.9137, 6.1554) -> (1.6405, 5.2892)
  line L436 (1.6405, 5.2892) -> (2.0296, 4.9)
  line L437 (2.0296, 4.9) -> (2.58, 4.9)
  line L438 (4.9, -2.58) -> (4.9985, -3.7064)
  line L439 (4.9985, -3.7064) -> (5.5365, -4.2635)
  line L440 (5.5365, -4.2635) -> (13.98, -12.4173)
  line L441 (13.98, -12.4173) -> (25.4085, -12.6168)
  line L442 (25.4085, -12.6168) -> (30.4597, -12.6168)
  line L443 (30.4597, -12.6168) -> (26.888, -9.0451)
  line L444 (26.888, -9.0451) -> (18.6658, -1.105)
  line L445 (18.6658, -1.105) -> (6.9296, -0.9001)
  line L446 (6.9296, -0.9001) -> (6.1554, -0.9137)
  line L447 (6.1554, -0.9137) -> (5.2892, -1.6405)
  line L448 (5.2892, -1.6405) -> (4.9, -2.0296)
  line L449 (4.9, -2.0296) -> (4.9, -2.58)
  line L450 (2.0296, -4.9) -> (1.6405, -5.2892)
  line L451 (1.6405, -5.2892) -> (0.9137, -6.1554)
  line L452 (0.9137, -6.1554) -> (0.9001, -6.9296)
  line L453 (0.9001, -6.9296) -> (1.105, -18.6658)
  line L454 (1.105, -18.6658) -> (9.0451, -26.888)
  line L455 (9.0451, -26.888) -> (12.6168, -30.4597)
  line L456 (12.6168, -30.4597) -> (12.6168, -25.4085)
  line L457 (12.6168, -25.4085) -> (12.4173, -13.98)
  line L458 (12.4173, -13.98) -> (4.2635, -5.5365)
  line L459 (4.2635, -5.5365) -> (3.7064, -4.9985)
  line L460 (3.7064, -4.9985) -> (2.58, -4.9)
  line L461 (2.58, -4.9) -> (2.0296, -4.9)
  line L462 (-15.6896, -14.4168) -> (-25.3928, -14.4168)
  line L463 (-25.3928, -14.4168) -> (-32.3817, -14.5388)
  line L464 (-32.3817, -14.5388) -> (-37.5003, -19.6574)
  line L465 (-37.5003, -19.6574) -> (-37.6102, -21.7546)
  line L466 (-37.6102, -21.7546) -> (-22.7683, -21.4955)
  line L467 (-22.7683, -21.4955) -> (-15.6896, -14.4168)
  line L468 (-30.4597, 12.6168) -> (-26.888, 9.0451)
  line L469 (-26.888, 9.0451) -> (-18.6658, 1.105)
  line L470 (-18.6658, 1.105) -> (-6.9296, 0.9001)
  line L471 (-6.9296, 0.9001) -> (-6.1554, 0.9137)
  line L472 (-6.1554, 0.9137) -> (-5.2892, 1.6405)
  line L473 (-5.2892, 1.6405) -> (-4.9, 2.0296)
  line L474 (-4.9, 2.0296) -> (-4.9, 2.58)
  line L475 (-4.9, 2.58) -> (-4.9985, 3.7064)
  line L476 (-4.9985, 3.7064) -> (-5.5365, 4.2635)
  line L477 (-5.5365, 4.2635) -> (-13.98, 12.4173)
  line L478 (-13.98, 12.4173) -> (-25.4085, 12.6168)
  line L479 (-25.4085, 12.6168) -> (-30.4597, 12.6168)
  circle A48 centre (0, 96.4395) radius 11.9225
  circle A49 centre (0, 96.4395) radius 7.5225
  dimension "d512" = 4.4
  constraint coincident L110.end L111.start
  constraint concentric A48 A49
  constraint coincident L111.end A48
  measures "d512" distance of A48 A49
extrude "Extrude4" add sketch "Sketch4" along normal up to surface (5 mm away) contours L110 L111 A48 A49 bodies 1